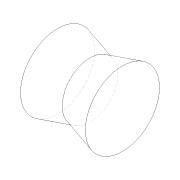
# Autodesk Inventor part: finger_thread_lock
Saved by Autodesk Inventor 2020.2 (Build 242310000, 310)
## iProperties
Created: 2020-04-09
Part Number: finger_thread_lock
Material: Generic
Document SubType Name: Modeling
Designer: Bardo91
Density: 1 g/cm^3
Appearance: Default
Author: Bardo91
Autodesk Inventor part; units mm, degrees
ref_plane "YZ Plane" through (0, 0, 0) normal (1, 0, 0) x (0, 1, 0)
ref_plane "XZ Plane" through (0, 0, 0) normal (0, 1, 0) x (-1, 0, 0)
ref_plane "XY Plane" through (0, 0, 0) normal (0, 0, 1) x (1, 0, 0)
sketch "Sketch1" plane through (0, 0, 0) normal (0, 0, 1) x (1, 0, 0)
  line L0 (0, 0) -> (1.75, 0)
  line L1 (1.75, 0) -> (1.75, 1)
  line L2 (0, 0) -> (0, 0.75)
  line L3 (0, 0.75) -> (1.75, 1)
  line L4 (0, 0) -> (-1.75, 0)
  line L5 (-1.75, 0) -> (-1.75, 1)
  line L6 (0, 0.75) -> (-1.75, 1)
  dimension "d0" = 1.75
  dimension "d1" = 1
  dimension "d2" = 0.75
  constraints: 14 end point, 2 symmetric about line, 2 vertical, 1 horizontal
  measures "d0" distance of L0.start L0.end
  measures "d1" distance of L0.end L1.end
  measures "d2" distance of L0.start L2.end
revolve "Revolution1" add sketch "Sketch1" angle 360 about axis through (0, 0, 0) along (1, 0, 0)
body "Solid1"
